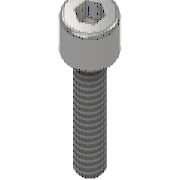
# Autodesk Inventor part: HexSocketCapScrew_M3x0.5-10
Saved by Autodesk Inventor 2024 (Build 280153000, 153)
## iProperties
Created: 2022-10-18
Part Number: HexSocketCapScrew_M3x0.5-10
Material: 鋼、軟鋼
Description: 六角穴付きボルト
Document SubType Name: Modeling
Designer: jwith
Manufacturer: Y.H.
Language: ja-JP
Categories: <MemberInstance><Categories><Category DisplayName="締結器具" InternalName="e4da775c-781d-43d5-af7c-5136215cf5a6" Mnemonic="FSTN"><Category DisplayName="ボルト" InternalName="536e6df0-f778-49ac-b2f2-25c71d2aa0b2" Mnemonic="SCRW"><CategoryParameter DisplayName="呼び径指定" InternalName="03caf894-eafd-4c09-a035-916ac084b87b" Mnemonic="nomdiadesig"/><CategoryParameter DisplayName="呼び長さ" InternalName="238ecbaf-3e6c-45dd-aa95-4068c8e0fd02" Mnemonic="nomlen"/><CategoryParameter DisplayName="ねじの名称" InternalName="586d5e89-370a-4089-914f-0110033585c7" Mnemonic="thrdesign"/><CategoryParameter DisplayName="ねじの種類の名称" InternalName="87c5849c-b3a5-4c3e-9c9b-2feecef9be86" Mnemonic="thrserdsgn"/><CategoryParameter DisplayName="呼び径" InternalName="8bbe3f8e-44cf-40a9-a251-3a6edc8168d6" Mnemonic="nomdia"/><CategoryParameter DisplayName="ねじの規格" InternalName="b4bbb7bc-d6aa-4c9f-a9a9-4152b9f6fe49" Mnemonic="thrtype"/><CategoryParameter DisplayName="ねじのピッチ" InternalName="bb82302e-82d8-4176-8fc1-c5d7bb17d5ad" Mnemonic="pitch1"/><CategoryParameter DisplayName="単位ごとのねじ" InternalName="bdc6e7d2-ffd0-4d9c-a173-16b95ebb912d" Mnemonic="thrperunit1"/><CategoryParameter DisplayName="ねじ等級" InternalName="ebc0d23b-2cc6-4d2a-b376-d52aae53bab6" Mnemonic="thrclss"/><Category DisplayName="穴付き" InternalName="55e06bf3-7e58-486c-bbdc-745fcc60664d" Mnemonic="CLSCRW"><CategoryParameter DisplayName="円筒部の呼び径" InternalName="179dbae3-102f-48bb-85fe-1e3ecd34f7cc" Mnemonic="grpdia"/><CategoryParameter DisplayName="ねじの長さ" InternalName="3268731d-5f9a-4750-8b01-4a959c46fbf2" Mnemonic="thrlen"/><CategoryParameter DisplayName="頭部の直径" InternalName="46177176-dbdd-4a1b-aefd-4c60c45016af" Mnemonic="headdia"/><CategoryParameter DisplayName="グリップ長さ" InternalName="52eab69f-422f-4795-9995-175a1b827e67" Mnemonic="grplen"/><CategoryParameter DisplayName="タイプ" InternalName="59a7e495-7a0c-4a5c-bdfd-c090c5f6e2db" Mnemonic="type"/><CategoryParameter DisplayName="頭部の高さ" InternalName="99c92c4c-4a02-4ebe-9e64-948fb169e19e" Mnemonic="headh"/></Category></Category></Category><Category DisplayName="データタイプ" InternalName="23b78d0f-2648-40c6-8793-ca6db495c9e8" Mnemonic="DATATYPE"><CategoryParameter DisplayName="表示名" InternalName="05415f3d-3907-474b-a020-eb9d644f4cf3" Mnemonic="DISPLAYNAME"/><CategoryParameter DisplayName="規格" InternalName="0c0a119c-1e12-4c84-803f-101930972f5e" Mnemonic="STANDARD"/><CategoryParameter DisplayName="説明" InternalName="13903e3d-64b1-4950-80da-f627842ea37f" Mnemonic="DESCRIPTION"/><CategoryParameter DisplayName="指定" InternalName="2675968c-4ce5-49e0-a4f5-552d29089031" Mnemonic="DESIGNATION"/><CategoryParameter DisplayName="既定行" InternalName="2af9ec52-faaa-4026-b378-f9fa4afca842" Mnemonic="DEFAULTROW"/><CategoryParameter DisplayName="フォルダ名" InternalName="3f06958e-8713-4116-9be7-ed6184ecc97b" Mnemonic="FOLDERNAME"/><CategoryParameter DisplayName="リビジョン ガイド" InternalName="45a75005-10b1-4dfc-8d6d-dfe629f0b93c" Mnemonic="REVISIONGUID"/><CategoryParameter DisplayName="ファイル名" InternalName="8b46a4cc-9585-4fed-90c3-899f57e09a73" Mnemonic="FILENAME"/><CategoryParameter DisplayName="標準化団体" InternalName="8f5914e1-4693-403f-8ab5-d37768198c9d" Mnemonic="STDSORG"/><CategoryParameter DisplayName="ファミリ バージョン" InternalName="914462f6-6e19-4b14-ba84-155b9680b1d0" Mnemonic="FAMILYREVISION"/><CategoryParameter DisplayName="規格のリビジョン" InternalName="91d5a463-65c2-4fde-b823-3b7fea5e8e17" Mnemonic="STANDARDREVISION"/><CategoryParameter DisplayName="メンバ履歴" InternalName="a65d44b9-392f-4f4f-857b-e4b3d54996fe" Mnemonic="MEMBERREVISION"/><CategoryParameter DisplayName="クリップ フォーマット" InternalName="bc51e27b-3422-4e78-93ef-cec197ddf230" Mnemonic="CLIPFORMAT"/><CategoryParameter DisplayName="製造者" InternalName="cd6c7a72-a28a-4e50-99a9-2c7f4e13e5ad" Mnemonic="MANUFACTURER"/><CategoryParameter DisplayName="内部名" InternalName="cf1d0246-76d9-4b4a-8305-fa0409afb5c1" Mnemonic="INTERNALNAME"/><CategoryParameter DisplayName="IsMetric" InternalName="e2385c5b-1ea4-4823-96a8-8de651266ec3" Mnemonic="ISMETRIC"/><Category DisplayName="パーツ" InternalName="c0e0b642-3bcb-4cc8-9e80-f96d35c4afa4" Mnemonic="PART"><CategoryParameter DisplayName="部品番号" InternalName="016b6077-bfbe-49bd-92c9-d8d59c39c941" Mnemonic="PARTNUMBER"/><CategoryParameter DisplayName="ストック番号" InternalName="4dba7c1c-e26c-444e-836c-b08b433409a8" Mnemonic="STOCKNUMBER"/><CategoryParameter DisplayName="材料キー" InternalName="5c9a8adb-dd2b-4535-b97f-0a94a95fe41f" Mnemonic="MATERIALKEY"/><CategoryParameter DisplayName="材料" InternalName="818a152a-d3c3-49ca-80ee-df7d91421b8e" Mnemonic="MATERIAL"/></Category></Category></Categories><FamilyTemplate Id="HexSocketCapScrew"><FamilyTemplateParameters><FamilyTemplateParameter ObjectType="kUserParameterObject" ValueType="xs:double" Id="12" ObjectReferenceKey="Pitch"/><FamilyTemplateParameter ObjectType="kUserParameterObject" ValueType="xs:double" Id="13" ObjectReferenceKey="NominalDiam"/><FamilyTemplateParameter ObjectType="kUserParameterObject" ValueType="xs:double" Id="14" ObjectReferenceKey="ThreadLength"/><FamilyTemplateParameter ObjectType="kUserParameterObject" ValueType="xs:double" Id="16" ObjectReferenceKey="HeadDiam"/><FamilyTemplateParameter ObjectType="kUserParameterObject" ValueType="xs:double" Id="17" ObjectReferenceKey="HeadHeight"/><FamilyTemplateParameter ObjectType="kUserParameterObject" ValueType="xs:double" Id="38" ObjectReferenceKey="SIZE_SEL"/><FamilyTemplateParameter ObjectType="kUserParameterObject" ValueType="xs:double" Id="66" ObjectReferenceKey="HeadFilletRad"/><FamilyTemplateParameter ObjectType="kUserParameterObject" ValueType="xs:double" Id="67" ObjectReferenceKey="NominalLength"/><FamilyTemplateParameter ObjectType="kUserParameterObject" ValueType="xs:double" Id="68" ObjectReferenceKey="RRad"/><FamilyTemplateParameter ObjectType="kUserParameterObject" ValueType="xs:double" Id="69" ObjectReferenceKey="SocketDepth"/><FamilyTemplateParameter ObjectType="kUserParameterObject" ValueType="xs:double" Id="70" ObjectReferenceKey="SocketWidth"/><FamilyTemplateParameter ObjectType="kPartComponentDefinitionObject" ValueType="xs:string" Id="49" SubObjectId="Material"/><FamilyTemplateParameter ObjectType="kPropertyObject" ValueType="xs:string" Id="59" ObjectReferenceKey="{32853F0F-3444-11d1-9E93-0060B03C1CA6}" SubObjectId="5"/><FamilyTemplateParameter ObjectType="kRenderStyleObject" ValueType="xs:string" Id="63" SubObjectId="RenderStyle"/><FamilyTemplateParameter ObjectType="kThreadFeatureObject" ValueType="xs:string" Id="71" ObjectReferenceKey="1002000010000000f00f0000000000008000000000000000" SubObjectId="ThreadInfo"><FamilyTemplateParameter ObjectType="" ValueType="xs:string" Id="72" SubObjectId="ThreadDesignation"/></FamilyTemplateParameter><FamilyTemplateParameter ObjectType="kPropertyObject" ValueType="xs:string" Id="75" ObjectReferenceKey="{D5CDD505-2E9C-101B-9397-08002B2CF9AE}" SubObjectId="Type"/></FamilyTemplateParameters></FamilyTemplate><CategoryParameterMap><ParamToTemplateMap><ParamToTemplate CategoryParameter="//CategoryParameter[@InternalName='cf1d0246-76d9-4b4a-8305-fa0409afb5c1']" ConstantValue="78ad96b8-146d-4ae5-870a-0abea777b22e"/><ParamToTemplate CategoryParameter="//CategoryParameter[@InternalName='45a75005-10b1-4dfc-8d6d-dfe629f0b93c']" ConstantValue="847f2713-dc09-4861-be83-79a551bc97c1"/><ParamToTemplate CategoryParameter="//CategoryParameter[@InternalName='3f06958e-8713-4116-9be7-ed6184ecc97b']" ConstantValue="HexSocketCapScrew"/><ParamToTemplate CategoryParameter="//CategoryParameter[@InternalName='8f5914e1-4693-403f-8ab5-d37768198c9d']" TemplateParameter="43"/><ParamToTemplate CategoryParameter="//CategoryParameter[@InternalName='0c0a119c-1e12-4c84-803f-101930972f5e']" TemplateParameter="44"/><ParamToTemplate CategoryParameter="//CategoryParameter[@InternalName='91d5a463-65c2-4fde-b823-3b7fea5e8e17']" TemplateParameter="45"/><ParamToTemplate CategoryParameter="//CategoryParameter[@InternalName='cd6c7a72-a28a-4e50-99a9-2c7f4e13e5ad']" ConstantValue="Y.H."/><ParamToTemplate CategoryParameter="//CategoryParameter[@InternalName='13903e3d-64b1-4950-80da-f627842ea37f']" ConstantValue="六角穴付きボルト"/><ParamToTemplate CategoryParameter="//CategoryParameter[@InternalName='05415f3d-3907-474b-a020-eb9d644f4cf3']" ConstantValue="HexSocketCapScrew"/><ParamToTemplate CategoryParameter="//CategoryParameter[@InternalName='914462f6-6e19-4b14-ba84-155b9680b1d0']" ConstantValue="11"/><ParamToTemplate CategoryParameter="//CategoryParameter[@InternalName='bc51e27b-3422-4e78-93ef-cec197ddf230']" ConstantValue="CF_INVENTOR.STDPARTS"/><ParamToTemplate CategoryParameter="//CategoryParameter[@InternalName='e2385c5b-1ea4-4823-96a8-8de651266ec3']" ConstantValue="true"/><ParamToTemplate CategoryParameter="//CategoryParameter[@InternalName='2af9ec52-faaa-4026-b378-f9fa4afca842']" ConstantValue="1"/><ParamToTemplate CategoryParameter="//CategoryParameter[@InternalName='ebc0d23b-2cc6-4d2a-b376-d52aae53bab6']" ConstantValue="6g"/><ParamToTemplate CategoryParameter="//CategoryParameter[@InternalName='8b46a4cc-9585-4fed-90c3-899f57e09a73']" ConstantValue="HexSocketCapScrew_3005010BK"/><ParamToTemplate CategoryParameter="//CategoryParameter[@InternalName='2675968c-4ce5-49e0-a4f5-552d29089031']" ConstantValue="M3x0.5-10"/><ParamToTemplate CategoryParameter="//CategoryParameter[@InternalName='a65d44b9-392f-4f4f-857b-e4b3d54996fe']" ConstantValue="f9c592e8-1bfc-4762-9476-f1662f12fda1"/><ParamToTemplate CategoryParameter="//CategoryParameter[@InternalName='52eab69f-422f-4795-9995-175a1b827e67']" ConstantValue="1.5"/><ParamToTemplate CategoryParameter="//CategoryParameter[@InternalName='a65d44b9-392f-4f4f-857b-e4b3d54996fe']" ConstantValue="f9c592e8-1bfc-4762-9476-f1662f12fda1"/><ParamToTemplate CategoryParameter="//CategoryParameter[@InternalName='87c5849c-b3a5-4c3e-9c9b-2feecef9be86']" ConstantValue="Regular Thread"/><ParamToTemplate CategoryParameter="//CategoryParameter[@InternalName='46177176-dbdd-4a1b-aefd-4c60c45016af']" TemplateParameter="16"/><ParamToTemplate CategoryParameter="//CategoryParameter[@InternalName='99c92c4c-4a02-4ebe-9e64-948fb169e19e']" TemplateParameter="17"/><ParamToTemplate CategoryParameter="//CategoryParameter[@InternalName='818a152a-d3c3-49ca-80ee-df7d91421b8e']" TemplateParameter="49"/><ParamToTemplate CategoryParameter="//CategoryParameter[@InternalName='8bbe3f8e-44cf-40a9-a251-3a6edc8168d6']" TemplateParameter="13"/><ParamToTemplate CategoryParameter="//CategoryParameter[@InternalName='238ecbaf-3e6c-45dd-aa95-4068c8e0fd02']" TemplateParameter="67"/><ParamToTemplate CategoryParameter="//CategoryParameter[@InternalName='016b6077-bfbe-49bd-92c9-d8d59c39c941']" TemplateParameter="59"/><ParamToTemplate CategoryParameter="//CategoryParameter[@InternalName='bb82302e-82d8-4176-8fc1-c5d7bb17d5ad']" TemplateParameter="12"/><ParamToTemplate CategoryParameter="//CategoryParameter[@InternalName='03caf894-eafd-4c09-a035-916ac084b87b']" TemplateParameter="38"/><ParamToTemplate CategoryParameter="//CategoryParameter[@InternalName='586d5e89-370a-4089-914f-0110033585c7']" TemplateParameter="72"/><ParamToTemplate CategoryParameter="//CategoryParameter[@InternalName='3268731d-5f9a-4750-8b01-4a959c46fbf2']" TemplateParameter="14"/></ParamToTemplateMap></CategoryParameterMap></MemberInstance>
Density: 7.85 g/cm^3
Appearance: 陽極酸化 - 黒
IsCustomPart: 0
Author: jwith
Type: HexSocketCapScrew
Autodesk Inventor part; units mm, degrees
ref_plane "YZ Plane" through (0, 0, 0) normal (1, 0, 0) x (0, 1, 0)
ref_plane "XZ Plane" through (0, 0, 0) normal (0, 1, 0) x (-1, 0, 0)
ref_plane "XY Plane" through (0, 0, 0) normal (0, 0, 1) x (1, 0, 0)
sketch "スケッチ1" plane through (0, 0, 0) normal (0, 1, 0) x (-1, 0, 0)
  line L0 (0, -10) -> (1.5, -10)
  line L1 (1.5, -10) -> (1.5, 0)
  line L2 (1.5, 0) -> (2.75, 0)
  line L3 (2.75, 0) -> (2.75, 3)
  line L4 (2.75, 3) -> (1.4434, 3)
  line L5 (1.4434, 1.7) -> (0, 0.8667)
  line L6 (0, 0.8667) -> (0, -10)
  line L7 (0, -12.6) -> (0, 5.6) projected
  line L8 (1.4434, 1.7) -> (1.4434, 3)
  point P0 (0, 0)
  dimension "nominaldiam" = 3
  dimension "nominallength" = 10
  dimension "headdiam" = 5.5
  dimension "headheight" = 3
  dimension "socketdiam" = 2.8868
  dimension "socketdepth" = 1.3
  dimension "socketangle" = 60
  constraints: 16 end point, 4 vertical, 3 horizontal, 2 point on line
  measures "nominaldiam" diameter of L1 L6
  measures "nominallength" distance between parallel lines of L0 L2
  measures "headdiam" diameter of L3 L6
  measures "headheight" distance between parallel lines of L4 L2
  measures "socketdiam" diameter of L4.end L6
  measures "socketdepth" distance of L5.start L4.end
  measures "socketangle" angle of L7 L5
revolve "ボディ" add sketch "スケッチ1" angle 360 about axis through (0, 0, 0.8667) along (0, 0, -1)
sketch "スケッチ2" plane through (0, 0, 3) normal (0, 0, 1) x (1, 0, 0)
  line L0 (0.7217, -1.25) -> (-0.7217, -1.25)
  line L1 (-0.7217, -1.25) -> (-1.4434, 0)
  line L2 (-1.4434, 0) -> (-0.7217, 1.25)
  line L3 (-0.7217, 1.25) -> (0.7217, 1.25)
  line L4 (0.7217, 1.25) -> (1.4434, 0)
  line L5 (1.4434, 0) -> (0.7217, -1.25)
  circle A0 centre (0, 0) radius 1.4434 projected
  point P0 (0, 0)
  point P1 (0, 0)
  point P2 (0.7217, -1.25)
  point P3 (0.7217, -1.25)
  point P4 (0.7217, 1.25)
  point P5 (0.7217, 1.25)
  point P6 (-0.7217, 1.25)
  point P7 (-0.7217, 1.25)
  point P8 (-1.4434, 0)
  point P9 (-1.4434, 0)
  point P10 (-0.7217, -1.25)
  point P11 (-0.7217, -1.25)
  constraints: 12 end point, 1 coincident, 1 horizontal alignment, 15 other
extrude "六角穴" add sketch "スケッチ2" against normal up to next contours A0 L0 | L5 A0 | A0 L1 | L4 A0 | A0 L2 | L3 A0
fillet "フィレット1" radius 0.3 1 edges at (2.75, 0, 3)
thread "ねじ1" size "M3x0.5" class "6g" standard "ISO Metric profile" length 8.5
chamfer "面取り1" distance 0.3067 distance2 0.3068 1 edges at (1.5, 0, -10) measured on face at (1, 0, -10)
fillet "フィレット2" radius 0.1 1 edges at (1.5, 0, 0)
equation "\"headfilletrad\" = HeadFilletRad"
equation "\"threadlength\" = ThreadLength"
equation "\"chamfer1\" = 0.61345 * Pitch"
equation "\"rrad\" = RRad"
equation "\"nominaldiam\" = NominalDiam"
equation "\"nominallength\" = NominalLength"
equation "\"headdiam\" = HeadDiam"
equation "\"headheight\" = HeadHeight"
equation "\"socketdiam\" = 1.1547 * SocketWidth"
equation "\"socketdepth\" = SocketDepth"
equation "\"NominalDiam\" = 3"
equation "\"NominalLength\" = 10"
equation "\"ThreadLength\" = 8.5"
equation "\"HeadDiam\" = 5.5"
equation "\"HeadHeight\" = 3"
equation "\"SocketWidth\" = 2.5"
equation "\"SocketDepth\" = 1.3"
equation "\"HeadFilletRad\" = 0.3"
equation "\"RRad\" = 0.1"
equation "\"Pitch\" = 0.5"
